DHECPVCdowelconnector (Autodesk Fusion 360 design; units mm, degrees)
Autodesk Fusion 360 part; units mm, degrees
note: some values were not read from the file. Set by a fixed rule: which sketch regions a step uses.
sketch "Sketch1" plane through (0, 0, 0) normal (0, 0, 1) x (1, 0, 0)
  circle A0 centre (0, 0) radius 45
  circle A1 centre (0, 0) radius 47
  dimension "d1" = 90
  dimension "d3" = 2
  constraint coincident A0.centre A1.centre
  measures "d1" diameter of A0
  measures "d3" distance of A0 A1
extrude "Extrude1" add sketch "Sketch1" along normal blind 16
ref_plane "WorkPlane1" through (55, 0, 0) normal (1, 0, 0) x (0, 1, 0)
sketch "Sketch2" plane through (55, 0, 0) normal (1, 0, 0) x (0, 1, 0)
  circle A0 centre (55, 8) radius 4.875
  circle A1 centre (55, 8) radius 8
  line L0 (47, 16) -> (-47, 16)
  line L1 (47, 0) -> (-47, 0)
  line L2 (47, 16) -> (55, 16)
  line L3 (47, 0) -> (55, 0)
  line L4 (47, 16) -> (42, 16)
  line L5 (42, 16) -> (42, 0)
  line L6 (42, 0) -> (47, 0)
  line L7 (47, 0) -> (47, 16)
  dimension "d7" = 9.75
  dimension "d10" = 5
  constraint tangent A1 L0
  constraint tangent A1 L1
  constraint concentric A0 A1
  constraint coincident L0.start L2.start
  constraint coincident A1 L2.end
  constraint tangent A1 L2
  constraint parallel L0 L2
  constraint coincident L1.start L3.start
  constraint coincident A1 L3.end
  constraint tangent A1 L3
  constraint parallel L1 L3
  constraint horizontal L4
  constraint vertical L5
  constraint horizontal L6
  constraint vertical L7
  constraint coincident L1 L5.end
  constraint tangent A1 L7
  measures "d7" diameter of A0
  measures "d10" distance of L5 L7
extrude "Extrude2" add sketch "Sketch2" along normal mid plane 40 from surface at -55
sketch "Sketch3" plane through (0, 0, 16) normal (0, 0, 1) x (-1, 0, 0)
  arc A0 (20, -42.5323) -> (-20, -42.5323) centre (0, 0) ccw
  line L0 (-20, -42.5323) -> (-20, -55)
  line L1 (-20, -55) -> (20, -55)
  line L2 (20, -55) -> (20, -42.5323)
  arc A1 (16.1555, -42) -> (-16.1555, -42) centre (0, 0) ccw
  line L3 (16.1555, -42) -> (-16.1555, -42)
  circle A2 centre (0, 0) radius 45
  line L4 (5, -50) -> (-5, -50)
  line L5 (-5, -50) -> (-5, -65)
  line L6 (-5, -65) -> (5, -65)
  line L7 (5, -65) -> (5, -50)
  dimension "d13" = 5
  dimension "d14" = 5
  dimension "d15" = 50
  dimension "d16" = 15
  constraint concentric A0 A2
  constraint horizontal L4
  constraint vertical L5
  constraint horizontal L6
  constraint vertical L7
  constraint coincident A1.end A2
  measures "d13" distance of A0.centre L7
  measures "d14" distance of A0.centre L5
  measures "d15" distance of A0.centre L4
  measures "d16" distance of L4 L6
extrude "Extrude3" cut sketch "Sketch3" against normal through all contours L1 L5 L6 L7 | L1 L4 L5 L7 | A1 L3 A2 | L3 A2
